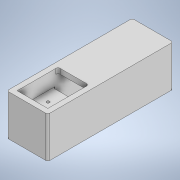
# Autodesk Inventor part: Link6_v2
Saved by Autodesk Inventor 2022 (Build 260153000, 153)
## iProperties
Created: 2022-06-14
Part Number: Link6_v2
Material: Generic
Document SubType Name: Modeling
Designer: Asus
Density: 1 g/cm^3
Appearance: Default
Author: Asus
Autodesk Inventor part; units mm, degrees
ref_plane "YZ Plane" through (0, 0, 0) normal (1, 0, 0) x (0, 1, 0)
ref_plane "XZ Plane" through (0, 0, 0) normal (0, 1, 0) x (-1, 0, 0)
ref_plane "XY Plane" through (0, 0, 0) normal (0, 0, 1) x (1, 0, 0)
sketch "Sketch1" plane through (0, 0, 0) normal (0, 1, 0) x (-1, 0, 0)
  line L0 (20, 22.5) -> (-20, 22.5)
  line L1 (-20, 22.5) -> (-20, -100)
  line L2 (-20, -100) -> (20, -100)
  line L3 (20, -100) -> (20, 22.5)
  circle A0 centre (0, 0) radius 4
  dimension "d0" = 122.5
  dimension "d1" = 22.5
  dimension "d2" = 40
  dimension "d3" = 20
  dimension "d4" = 8
  constraints: 8 end point, 2 parallel, 1 centre point, 1 coincident, 1 horizontal, 1 perpendicular
  measures "d0" distance of L0.end L1.end
  measures "d1" distance from line of point (0, 0) L0
  measures "d2" distance of L0.start L0.end
  measures "d3" distance from line of L3 point (0, 0)
  measures "d4" diameter of A0
extrude "Extrusion1" add sketch "Sketch1" along normal blind 5
sketch "Sketch2" plane through (0, 5, 0) normal (0, 1, 0) x (1, 0, 0)
  line L0 (-20, 100) -> (-20, -22.5) projected
  line L1 (20, -22.5) -> (20, 100) projected
  line L2 (-20, -22.5) -> (20, -22.5)
  line L3 (20, -22.5) -> (20, 100)
  line L4 (20, 100) -> (-20, 100)
  line L5 (-20, 100) -> (-20, -22.5)
  line L6 (-15, -17.5) -> (15, -17.5)
  line L7 (15, -17.5) -> (15, 95)
  line L8 (15, 95) -> (-15, 95)
  line L9 (-15, 95) -> (-15, -17.5)
  point P0 (0, 0)
  dimension "d7" = 5
  dimension "d8" = 5
  dimension "d9" = 5
  dimension "d10" = 5
  constraints: 16 end point, 4 parallel, 2 horizontal, 2 perpendicular
  measures "d7" distance between parallel lines of L4 L8
  measures "d8" distance between parallel lines of L7 L3
  measures "d9" distance between parallel lines of L0 L9
  measures "d10" distance between parallel lines of L2 L6
extrude "Extrusion2" add sketch "Sketch2" along normal blind 35
sketch "Sketch3" plane through (0, 40, 0) normal (0, 1, 0) x (1, 0, 0)
  line L0 (-20, 100) -> (-20, -22.5) projected
  line L1 (20, -22.5) -> (20, 100) projected
  line L2 (-20, 100) -> (20, 100)
  line L3 (20, 100) -> (20, 22.5)
  line L4 (20, 22.5) -> (-20, 22.5)
  line L5 (-20, 22.5) -> (-20, 100)
  point P0 (0, 0)
  point P1 (-20, 22.5)
  dimension "d13" = 77.5
  constraints: 8 end point, 2 parallel, 1 horizontal, 1 perpendicular, 1 point on line
  measures "d13" distance between parallel lines of L2 L4
extrude "Extrusion3" add sketch "Sketch3" against normal blind 5
sketch "Sketch4" plane through (0, 5, 0) normal (0, 1, 0) x (1, 0, 0)
  line L0 (-15, -17.5) -> (-15, 22.5) projected
  line L1 (15, 22.5) -> (15, -17.5) projected
  line L2 (-15, -17.5) -> (15, -17.5)
  line L3 (15, -17.5) -> (15, 17.5)
  line L4 (15, 17.5) -> (-15, 17.5)
  line L5 (-15, 17.5) -> (-15, -17.5)
  point P0 (0, 0)
  point P1 (-15, 17.5)
  dimension "d16" = 35
  constraints: 8 end point, 2 parallel, 1 horizontal, 1 perpendicular, 1 point on line
  measures "d16" distance between parallel lines of L2 L4
extrude "Extrusion4" add sketch "Sketch4" along normal blind 20
sketch "Sketch5" plane through (0, 0, 0) normal (0, -1, 0) x (1, 0, 0)
  circle A0 centre (0, 0) radius 4 projected
  circle A1 centre (0, 0) radius 9.5
  dimension "d19" = 19
  constraints: 1 centre point, 1 coincident
  measures "d19" diameter of A1
extrude "Extrusion5" cut sketch "Sketch5" against normal blind 12.5 contours A0 | A1
sketch "Sketch6" plane through (0, 0, 0) normal (0, -1, 0) x (1, 0, 0)
  circle A0 centre (0, 0) radius 11.5
  dimension "d22" = 23
  constraints: 1 centre point, 1 coincident
  measures "d22" diameter of A0
extrude "Extrusion6" cut sketch "Sketch6" against normal blind 6.5
sketch "Sketch7" plane through (0, 12.5, 0) normal (0, -1, 0) x (1, 0, 0)
  circle A0 centre (0, 0) radius 9.5 projected
  circle A1 centre (0, 0) radius 6.2
  line L0 (0, 0) -> (0, 7.0938)
  line L1 (0, 0) -> (7.0405, -4.0648)
  line L2 (0, 0) -> (-6.9896, -4.0354)
  circle A2 centre (0, 6.2) radius 1.45
  circle A3 centre (5.3694, -3.1) radius 1.45
  circle A4 centre (-5.3694, -3.1) radius 1.45
  dimension "d25" = 12.4
  dimension "d26" = 120
  dimension "d27" = 120
  dimension "d28" = 2.9
  dimension "d29" = 2.9
  dimension "d30" = 2.9
  constraints: 6 end point, 4 centre point, 3 point on circle, 3 point on line, 1 coincident, 1 vertical
  measures "d25" diameter of A1
  measures "d26" angle of L0 L2
  measures "d27" angle of L1 L2
  measures "d28" diameter of A3
  measures "d29" diameter of A4
  measures "d30" diameter of A2
extrude "Extrusion7" cut sketch "Sketch7" against normal blind 18 contours A2 L0 A1 | A1 A2 | A3 L1 A1 | A1 L1 A3 | L0 A2 A1 | L1 A3 A1 | A1 A3 L1 | A4 L2 A1 | A1 L2 A4 | A4 A1 L2 | A4 L2 A1
sketch "Sketch8" plane through (0, 0, 0) normal (0, -1, 0) x (1, 0, 0)
  line L0 (15, -95) -> (-15, -95) projected
  line L1 (-15, -95) -> (-15, -22.5) projected
  line L2 (15, -95) -> (-15, -95)
  line L3 (-15, -95) -> (-15, -17.5)
  line L4 (-15, -17.5) -> (15, -17.5)
  line L5 (15, -17.5) -> (15, -95)
  point P0 (0, 0)
  dimension "d33" = 77.5
  constraints: 8 end point, 2 parallel, 1 horizontal, 1 perpendicular, 1 point on line
  measures "d33" distance between parallel lines of L0 L4
extrude "Extrusion8" cut sketch "Sketch8" against normal blind 18
sketch "Sketch9" plane through (-15, 0, -95) normal (0, 0, 1) x (1, 0, 0)
  line L0 (30, 35) -> (0, 35) projected
  line L1 (30, 35) -> (0, 35)
  line L2 (0, 35) -> (0, 0)
  line L3 (0, 0) -> (30, 0)
  line L4 (30, 0) -> (30, 35)
  point P0 (15, 0)
  constraints: 8 end point, 2 parallel, 1 horizontal, 1 perpendicular
extrude "Extrusion9" add sketch "Sketch9" along normal blind 3
sketch "Sketch10" plane through (20, 0, -100) normal (0, 0, -1) x (-1, 0, 0)
  circle A0 centre (20, 20) radius 4
  line L0 (0, 0) -> (0, 40) projected
  line L1 (0, 0) -> (40, 0) projected
  line L2 (35, 35) -> (5, 35) projected
  line L3 (20, 35) -> (20, 7.5388)
  circle A1 centre (20, 20) radius 8.5
  circle A2 centre (20, 11.5) radius 1.5
  circle A3 centre (20, 28.5) radius 1.5
  point P0 (20, 0)
  dimension "d38" = 20
  dimension "d39" = 20
  dimension "d40" = 8
  dimension "d41" = 17
  dimension "d42" = 3
  dimension "d43" = 3
  constraints: 4 centre point, 2 end point, 2 point on circle, 2 point on line, 1 coincident, 1 midpoint, 1 perpendicular
  measures "d38" distance from line of L0 A0.centre
  measures "d39" distance from line of L1 A0.centre
  measures "d40" diameter of A0
  measures "d41" diameter of A1
  measures "d42" diameter of A2
  measures "d43" diameter of A3
extrude "Extrusion10" cut sketch "Sketch10" against normal blind 9 contours A0 L3 | L3 A0 | A3 A1 L3 | L3 A1 A3 | A2 A1 L3 | L3 A1 A2 | A1 A3 L3 | L3 A3 A1 | A1 A2 L3 | L3 A2 A1
fillet "Fillet1" radius 2 4 edges at (-20, 20, 22.5) (20, 20, 22.5) (20, 20, -100) (-20, 20, -100)
fillet "Fillet2" radius 2 2 edges at (15, 12.5, -17.5) (-15, 12.5, -17.5)
fillet "Fillet3" radius 2 2 edges at (-15, 37.5, -22.5) (15, 37.5, -22.5)
sketch "Sketch11" plane through (-15, 0, -92) normal (0, 0, 1) x (1, 0, 0)
  circle A0 centre (15, 20) radius 4 projected
  circle A1 centre (15, 20) radius 13
  point P0 (15, 0)
  dimension "d49" = 26
  constraints: 1 centre point, 1 coincident
  measures "d49" diameter of A1
extrude "Extrusion11" cut sketch "Sketch11" against normal blind 4
body "Solid1"
